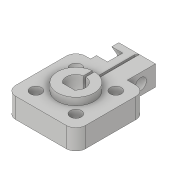
# Autodesk Inventor part: clamping hub 1_4 D nut wells
Saved by Autodesk Inventor 2020 (Build 240168000, 168)
## iProperties
Created: 2019-10-18
Part Number: clamping hub 1_4 D nut wells
Material: Generic
Document SubType Name: Modeling
Designer: ball
Density: 1 g/cm^3
Appearance: Default
Author: ball
Autodesk Inventor part; units mm, degrees
ref_plane "YZ Plane" through (0, 0, 0) normal (1, 0, 0) x (0, 1, 0)
ref_plane "XZ Plane" through (0, 0, 0) normal (0, 1, 0) x (-1, 0, 0)
ref_plane "XY Plane" through (0, 0, 0) normal (0, 0, 1) x (1, 0, 0)
sketch "Sketch1" plane through (0, 0, 0) normal (0, 1, 0) x (-1, 0, 0)
  line L0 (-12.065, 12.065) -> (12.065, 12.065)
  line L1 (12.065, 12.065) -> (12.065, -12.065)
  line L2 (-12.065, -12.065) -> (-12.065, 12.065)
  circle A0 centre (6.9148, -6.9148) radius 1.9304
  circle A1 centre (6.9148, 6.9148) radius 1.9304
  circle A2 centre (-6.9148, 6.9148) radius 1.9304
  circle A3 centre (-6.9148, -6.9148) radius 1.9304
  line L3 (-5.715, -12.065) -> (-5.715, -21.844)
  line L4 (-5.715, -21.844) -> (6.985, -21.844)
  line L5 (6.985, -21.844) -> (6.985, -12.065)
  line L6 (12.065, -12.065) -> (6.985, -12.065)
  line L7 (-5.715, -12.065) -> (-12.065, -12.065)
  point P0 (0, 0)
  dimension "d0" = 24.13
  dimension "d2" = 12.065
  dimension "d3" = 12.065
  dimension "d4" = 3.8608
  dimension "d5" = 6.9148
  dimension "d6" = 6.9148
  dimension "d7" = 3.8608
  dimension "d8" = 6.9148
  dimension "d9" = 6.9148
  dimension "d10" = 3.8608
  dimension "d11" = 6.9148
  dimension "d12" = 6.9148
  dimension "d13" = 3.8608
  dimension "d14" = 12.7
  dimension "d16" = 6.985
  dimension "d41" = 6.9148
  dimension "d42" = 6.9148
  dimension "d43" = 24.13
  dimension "d44" = 24.13
  dimension "d50" = 9.779
  dimension "d51" = 9.779
  constraints: 16 end point, 4 centre point, 4 parallel, 1 horizontal, 1 perpendicular
  measures "d0" distance of L1.end L2.start
  measures "d2" distance from line of L0 point (0, 0)
  measures "d3" distance from line of L1 point (0, 0)
  measures "d4" diameter of A0
  measures "d5" horizontal distance of A0.centre point (0, 0)
  measures "d6" horizontal distance of A0.centre point (0, 0)
  measures "d7" diameter of A1
  measures "d8" horizontal distance of point (0, 0) A1.centre
  measures "d9" horizontal distance of point (0, 0) A1.centre
  measures "d10" diameter of A2
  measures "d11" horizontal distance of point (0, 0) A2.centre
  measures "d12" horizontal distance of A2.centre point (0, 0)
  measures "d13" diameter of A3
  measures "d14" distance of L4.end L3.end
  measures "d16" distance from line of L5 point (0, 0)
  measures "d41" horizontal distance of A3.centre point (0, 0)
  measures "d42" horizontal distance of A3.centre point (0, 0)
  measures "d43" distance between parallel lines of L7 L0
  measures "d44" distance between parallel lines of L6 L0
  measures "d50" distance between parallel lines of L7 L4
  measures "d51" distance between parallel lines of L6 L4
extrude "Shape" add sketch "Sketch1" along normal blind 6.985
sketch "Sketch2" plane through (-6.985, 0, -21.844) normal (-1, 0, 0) x (0, 0, 1)
  circle A0 centre (5.08, 3.4925) radius 4.6609 construction
  line L0 (9.779, 0) -> (0, 0) projected
  line L1 (0, 0) -> (0, 6.985) projected
  line L2 (9.7409, 3.4925) -> (7.4105, -0.544)
  line L3 (7.4105, -0.544) -> (2.7496, -0.544)
  line L4 (2.7496, -0.544) -> (0.4191, 3.4925)
  line L5 (0.4191, 3.4925) -> (2.7495, 7.529)
  line L6 (2.7495, 7.529) -> (7.4104, 7.529)
  line L7 (7.4104, 7.529) -> (9.7409, 3.4925)
  line L8 (9.779, 0) -> (9.779, 6.985) projected
  point P0 (21.844, 0)
  dimension "d19" = 9.3218
  dimension "d20" = 3.4925
  dimension "d52" = 4.699
  constraints: 12 end point, 1 coincident, 1 horizontal alignment, 15 other
  measures "d20" distance from line of L0 point (5.08, 3.493)
  measures "d52" distance from line of L8 point (5.08, 3.493)
extrude "NutWellSide" cut sketch "Sketch2" against normal blind 3.81
sketch "Sketch3" plane through (5.715, 0, -12.065) normal (1, 0, 0) x (0, 0, -1)
  circle A0 centre (4.699, 3.4925) radius 1.9304
  line L0 (9.779, 0) -> (9.779, 6.985) projected
  line L1 (0, 6.985) -> (9.779, 6.985) projected
  line L2 (0, 0) -> (0, 6.985) projected
  point P0 (-12.065, 0)
  dimension "d24" = 3.8608
  dimension "d26" = 3.4925
  dimension "d53" = 4.699
  constraints: 1 centre point
  measures "d24" diameter of A0
  measures "d26" distance from line of L1 A0.centre
  measures "d53" distance from line of L2 A0.centre
extrude "HoleClamping" cut sketch "Sketch3" against normal through all
sketch "Sketch4" plane through (0, 6.985, 0) normal (0, 1, 0) x (1, 0, 0)
  circle A0 centre (0, 0) radius 6.35
  dimension "d29" = 12.7
  constraints: 1 centre point, 1 coincident
  measures "d29" diameter of A0
extrude "Boss" add sketch "Sketch4" along normal blind 2.54
sketch "Sketch5" plane through (0, 9.525, 0) normal (0, 1, 0) x (1, 0, 0)
  arc A0 (2.0472, -2.5908) -> (-2.0472, -2.5908) centre (0, 0) ccw
  line L0 (-2.0472, -2.5908) -> (2.0472, -2.5908)
  dimension "d32" = 6.604
  dimension "d33" = 2.5908
  constraints: 2 end point, 2 point on circle, 1 centre point, 1 coincident, 1 horizontal
  measures "d32" diameter of A0
  measures "d33" distance from line of L0 point (0, 0)
fillet "Fillet1" radius 3.3782 4 edges at (12.065, 3.4925, 12.065) (12.065, 3.4925, -12.065) (-12.065, 3.4925, 12.065) (-12.065, 3.4925, -12.065)
extrude "HoleD" cut sketch "Sketch5" against normal through all
sketch "Sketch6" plane through (0, 9.525, 0) normal (0, 1, 0) x (1, 0, 0)
  line L0 (-6.985, 21.844) -> (5.715, 21.844) projected
  line L1 (0.127, 0.254) -> (0.127, 21.844)
  line L2 (0.127, 21.844) -> (-0.635, 20.828)
  line L3 (-0.635, 20.828) -> (-0.635, 0.254)
  line L4 (-0.1123, -19.3229) -> (0.127, 21.844) construction
  line L5 (0.6195, -20.3205) -> (-0.635, 20.828) construction
  line L6 (-0.635, 0.254) -> (0.127, 0.254)
  point P0 (0, 0)
  dimension "d37" = 1.27
  constraints: 12 end point, 3 point on line, 1 parallel
  measures "d37" distance of L2.end L1.end
extrude "ClampingSlot" cut sketch "Sketch6" against normal through all
sketch "Sketch7" plane through (0, 0, 0) normal (0, -1, 0) x (1, 0, 0)
  circle A0 centre (-6.9148, 6.9148) radius 1.9304 construction
  circle A1 centre (-6.9148, 6.9148) radius 4.6609 construction
  line L0 (-6.9148, 2.2539) -> (-10.9513, 4.5843)
  line L1 (-10.9513, 4.5843) -> (-10.9513, 9.2452)
  line L2 (-10.9513, 9.2452) -> (-6.9148, 11.5757)
  line L3 (-6.9148, 11.5757) -> (-2.8783, 9.2452)
  line L4 (-2.8783, 9.2452) -> (-2.8783, 4.5843)
  line L5 (-2.8783, 4.5843) -> (-6.9148, 2.2539)
  circle A2 centre (-6.9148, -6.9148) radius 1.9304 construction
  circle A3 centre (-6.9148, -6.9148) radius 4.6609 construction
  circle A4 centre (6.9148, -6.9148) radius 1.9304 construction
  circle A5 centre (6.9148, -6.9148) radius 4.6609 construction
  circle A6 centre (6.9148, 6.9148) radius 1.9304 construction
  circle A7 centre (6.9148, 6.9148) radius 4.6609 construction
  line L6 (6.9148, 2.2539) -> (2.8783, 4.5843)
  line L7 (2.8783, 4.5843) -> (2.8783, 9.2452)
  line L8 (2.8783, 9.2452) -> (6.9148, 11.5757)
  line L9 (6.9148, 11.5757) -> (10.9513, 9.2452)
  line L10 (10.9513, 9.2452) -> (10.9513, 4.5843)
  line L11 (10.9513, 4.5843) -> (6.9148, 2.2539)
  line L12 (6.9148, -2.2539) -> (10.9513, -4.5843)
  line L13 (10.9513, -4.5843) -> (10.9513, -9.2452)
  line L14 (10.9513, -9.2452) -> (6.9148, -11.5757)
  line L15 (6.9148, -11.5757) -> (2.8783, -9.2452)
  line L16 (2.8783, -9.2452) -> (2.8783, -4.5843)
  line L17 (2.8783, -4.5843) -> (6.9148, -2.2539)
  line L18 (-6.9148, -2.2539) -> (-2.8783, -4.5843)
  line L19 (-2.8783, -4.5843) -> (-2.8783, -9.2452)
  line L20 (-2.8783, -9.2452) -> (-6.9148, -11.5757)
  line L21 (-6.9148, -11.5757) -> (-10.9513, -9.2452)
  line L22 (-10.9513, -9.2452) -> (-10.9513, -4.5843)
  line L23 (-10.9513, -4.5843) -> (-6.9148, -2.2539)
  point P0 (0, 0)
  dimension "d40" = 9.3218
  dimension "d45" = 9.3218
  dimension "d46" = 9.3218
  dimension "d47" = 9.3218
  constraints: 48 end point, 8 coincident, 4 vertical alignment, 60 other
extrude "NutWellAttachment" cut sketch "Sketch7" against normal blind 3.048
equation "\"d2\" = 0.5 * d0"
equation "\"d3\" = 0.5 * d0"
equation "\"d6\" = d9"
equation "\"d7\" = d4"
equation "\"d8\" = d9"
equation "\"d9\" = d5"
equation "\"d10\" = d4"
equation "\"d11\" = d9"
equation "\"d12\" = d9"
equation "\"d13\" = d4"
equation "\"d41\" = d9"
equation "\"d42\" = d5"
equation "\"d43\" = d0"
equation "\"d44\" = d0"
body "Solid1"
